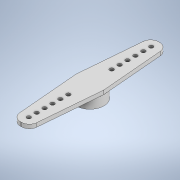
# Autodesk Inventor part: horn
Saved by Autodesk Inventor 2022 (Build 260153000, 153)
## iProperties
Created: 2023-04-19
Part Number: horn
Material: Generisch
Document SubType Name: Modeling
Designer: marti
Density: 1 g/cm^3
Appearance: Vorgabe
Author: marti
Autodesk Inventor part; units mm, degrees
ref_plane "YZ Plane" through (0, 0, 0) normal (1, 0, 0) x (0, 1, 0)
ref_plane "XZ Plane" through (0, 0, 0) normal (0, 1, 0) x (-1, 0, 0)
ref_plane "XY Plane" through (0, 0, 0) normal (0, 0, 1) x (1, 0, 0)
sketch "Skizze1" plane through (0, 0, 0) normal (0, 1, 0) x (-1, 0, 0)
  circle A0 centre (0, 0) radius 1.75
  circle A1 centre (0, 0) radius 3.5
  dimension "d2" = 3.5
  dimension "d3" = 7
  constraints: 2 centre point, 2 coincident
  measures "d2" diameter of A0
  measures "d3" diameter of A1
extrude "Extrusion1" add sketch "Skizze1" along normal blind 2.5
sketch "Skizze2" plane through (0, 2.5, 0) normal (0, 1, 0) x (1, 0, 0)
  line L0 (-2, 17.5) -> (2, 17.5)
  line L1 (2, 17.5) -> (2, -17.5)
  line L2 (2, -17.5) -> (-2, -17.5)
  line L3 (-2, -17.5) -> (-2, 17.5)
  line L4 (-2, 17.5) -> (2, -17.5) construction
  line L5 (2, 17.5) -> (-2, -17.5) construction
  circle A0 centre (0, 0) radius 3.5 projected
  line L6 (3.5, 0) -> (2, -17.5)
  line L7 (-2, -17.5) -> (-3.5, 0)
  circle A1 centre (0, 0) radius 3.5 projected
  line L8 (-3.5, 0) -> (-2, 17.5)
  line L9 (2, 17.5) -> (3.5, 0)
  dimension "d6" = 35
  dimension "d7" = 4
  constraints: 20 end point, 4 parallel, 2 midpoint, 1 horizontal, 1 horizontal alignment, 1 perpendicular, 1 point on circle, 1 other
  measures "d6" distance of L0.end L1.end
  measures "d7" distance of L0.start L0.end
extrude "Extrusion2" add sketch "Skizze2" along normal blind 1 contours L0 L1 A0 L3 | L3 A0 L8 | L9 A0 L1 | A0 L1 L3 | L3 A0 L7 L8 | A0 L9 L6 L1 | A0 L1 L2 L3 | L3 L7 A0 | A0 L6 L1
sketch "Skizze3" plane through (0, 3.5, 0) normal (0, 1, 0) x (1, 0, 0)
  line L0 (-2, -17.5) -> (2, -17.5) projected
  point P0 (0, 0)
  point P1 (0, -15.5)
  point P2 (0, -13.5)
  point P3 (0, -11.5)
  point P4 (0, -9.5)
  point P5 (0, -7.5)
  point P6 (0, -5.5)
  point P7 (0, 5.5)
  point P8 (0, 7.5)
  point P9 (0, 9.5)
  point P10 (0, 11.5)
  point P11 (0, 13.5)
  point P12 (0, 15.5)
  dimension "d10" = 2
  dimension "d11" = 2
  dimension "d12" = 2
  dimension "d13" = 2
  dimension "d14" = 2
  dimension "d15" = 2
  dimension "d16" = 0
  dimension "d17" = 0
  dimension "d18" = 2
  dimension "d19" = 2
  dimension "d20" = 2
  dimension "d21" = 2
  dimension "d22" = 2
  dimension "d24" = 5.5
  measures "d10" distance of point (0, -15.5) point (0, -13.5)
  measures "d11" distance of point (0, -5.5) point (0, -7.5)
  measures "d12" distance of point (0, -7.5) point (0, -9.5)
  measures "d13" distance of point (0, -9.5) point (0, -11.5)
  measures "d14" distance of point (0, -11.5) point (0, -13.5)
  measures "d15" distance from line of L0 point (0, -15.5)
  measures "d16" horizontal distance of point (0, 0) point (0, -15.5)
  measures "d17" horizontal distance of point (0, 0) point (0, -13.5)
  measures "d18" distance of point (0, 7.5) point (0, 5.5)
  measures "d19" distance of point (0, 9.5) point (0, 7.5)
  measures "d20" distance of point (0, 9.5) point (0, 11.5)
  measures "d21" distance of point (0, 11.5) point (0, 13.5)
  measures "d22" distance of point (0, 13.5) point (0, 15.5)
  measures "d24" distance of point (0, 5.5) point (0, 0)
hole "Bohrung1" at (0, 3.5, 15.5) at (0, 3.5, 13.5) at (0, 3.5, 11.5) at (0, 3.5, 9.5) at (0, 3.5, 7.5) at (0, 3.5, 5.5) at (0, 3.5, -5.5) at (0, 3.5, -7.5) at (0, 3.5, -9.5) at (0, 3.5, -11.5) at (0, 3.5, -13.5) at (0, 3.5, -15.5) direction (0, -1, 0) diameter 1 depth 8 tip angle 118
fillet "Rundung1" radius 2 4 edges at (2, 3, 17.5) (-2, 3, 17.5) (2, 3, -17.5) (-2, 3, -17.5)
